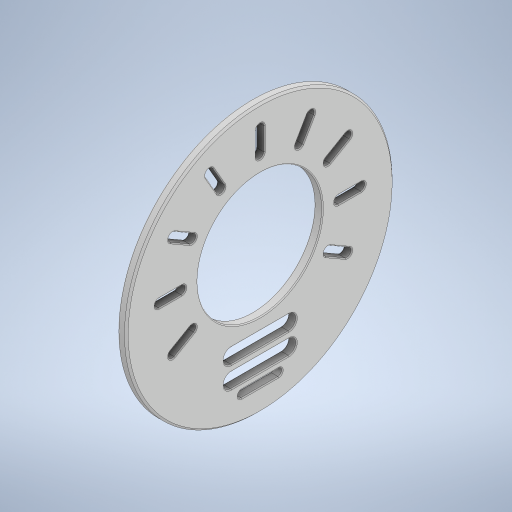
# Autodesk Inventor part: BacklightCaseFrontSymbolDisc
Saved by Autodesk Inventor 2023 (Build 270158000, 158)
## iProperties
Created: 2026-01-27
Part Number: BacklightCaseFrontSymbolDisc
Material: Generic
Document SubType Name: Modeling
Designer: DanAr
Density: 1 g/cm^3
Appearance: Default
Author: DanAr
Autodesk Inventor part; units mm, degrees
ref_plane "YZ Plane" through (0, 0, 0) normal (1, 0, 0) x (0, 1, 0)
ref_plane "XZ Plane" through (0, 0, 0) normal (0, 1, 0) x (-1, 0, 0)
ref_plane "XY Plane" through (0, 0, 0) normal (0, 0, 1) x (1, 0, 0)
sketch "Sketch1" plane through (0, 0, 0) normal (1, 0, 0) x (0, 1, 0)
  arc A0 (4.9525, -3.697) -> (-4.9525, -3.697) centre (0, 1.25) ccw
  circle A1 centre (0, 1.25) radius 6.5
  arc A2 (0.5, 12.2) -> (-0.5, 12.2) centre (0, 12.2) ccw
  arc A3 (-0.2, 9.75) -> (0.2, 9.75) centre (0, 9.75) ccw
  line L0 (0, 12.2) -> (0, 9.75) construction
  line L1 (-0.4, 12.2) -> (-0.4, 9.75)
  line L2 (0.4, 9.75) -> (0.4, 12.2)
  arc A4 (0.4, 12.2) -> (-0.4, 12.2) centre (0, 12.2) ccw
  arc A5 (-0.4, 9.75) -> (0.4, 9.75) centre (0, 9.75) ccw
  arc A6 (4.7402, -3.485) -> (-4.7403, -3.485) centre (0, 1.25) ccw
  circle A7 centre (0, 1.25) radius 10.95
  circle A8 centre (0, 1.25) radius 8.5
  circle A9 centre (0, 1.25) radius 11.35
  arc A10 (-5.3018, 10.833) -> (-5.6482, 10.633) centre (-5.475, 10.733) ccw
  arc A11 (-4.4232, 8.5112) -> (-4.0768, 8.7112) centre (-4.25, 8.6112) ccw
  line L3 (-5.475, 10.733) -> (-4.25, 8.6112) construction
  line L4 (-5.8214, 10.533) -> (-4.5964, 8.4112)
  line L5 (-3.9036, 8.8112) -> (-5.1286, 10.933)
  arc A12 (-5.1286, 10.933) -> (-5.8214, 10.533) centre (-5.475, 10.733) ccw
  arc A13 (-4.5964, 8.4112) -> (-3.9036, 8.8112) centre (-4.25, 8.6112) ccw
  arc A14 (-9.383, 6.8982) -> (-9.583, 6.5518) centre (-9.483, 6.725) ccw
  arc A15 (-7.4612, 5.3268) -> (-7.2612, 5.6732) centre (-7.3612, 5.5) ccw
  line L6 (-9.483, 6.725) -> (-7.3612, 5.5) construction
  line L7 (-9.683, 6.3786) -> (-7.5612, 5.1536)
  line L8 (-7.1612, 5.8464) -> (-9.283, 7.0714)
  arc A16 (-9.283, 7.0714) -> (-9.683, 6.3786) centre (-9.483, 6.725) ccw
  arc A17 (-7.5612, 5.1536) -> (-7.1612, 5.8464) centre (-7.3612, 5.5) ccw
  arc A18 (-10.95, 1.45) -> (-10.95, 1.05) centre (-10.95, 1.25) ccw
  arc A19 (-8.5, 1.05) -> (-8.5, 1.45) centre (-8.5, 1.25) ccw
  line L9 (-10.95, 1.25) -> (-8.5, 1.25) construction
  line L10 (-10.95, 0.85) -> (-8.5, 0.85)
  line L11 (-8.5, 1.65) -> (-10.95, 1.65)
  arc A20 (-10.95, 1.65) -> (-10.95, 0.85) centre (-10.95, 1.25) ccw
  arc A21 (-8.5, 0.85) -> (-8.5, 1.65) centre (-8.5, 1.25) ccw
  arc A22 (-7.2612, -3.1732) -> (-7.4612, -2.8268) centre (-7.3612, -3) ccw
  arc A23 (-9.583, -4.0518) -> (-9.383, -4.3982) centre (-9.483, -4.225) ccw
  line L12 (-7.3612, -3) -> (-9.483, -4.225) construction
  line L13 (-7.5612, -2.6536) -> (-9.683, -3.8786)
  line L14 (-9.283, -4.5714) -> (-7.1612, -3.3464)
  arc A24 (-7.1612, -3.3464) -> (-7.5612, -2.6536) centre (-7.3612, -3) ccw
  arc A25 (-9.683, -3.8786) -> (-9.283, -4.5714) centre (-9.483, -4.225) ccw
  arc A26 (4.0768, 8.7112) -> (4.4232, 8.5112) centre (4.25, 8.6112) ccw
  arc A27 (5.6482, 10.633) -> (5.3018, 10.833) centre (5.475, 10.733) ccw
  line L15 (4.25, 8.6112) -> (5.475, 10.733) construction
  line L16 (4.5964, 8.4112) -> (5.8214, 10.533)
  line L17 (5.1286, 10.933) -> (3.9036, 8.8112)
  arc A28 (3.9036, 8.8112) -> (4.5964, 8.4112) centre (4.25, 8.6112) ccw
  arc A29 (5.8214, 10.533) -> (5.1286, 10.933) centre (5.475, 10.733) ccw
  arc A30 (7.2612, 5.6732) -> (7.4612, 5.3268) centre (7.3612, 5.5) ccw
  arc A31 (9.583, 6.5518) -> (9.383, 6.8982) centre (9.483, 6.725) ccw
  line L18 (7.3612, 5.5) -> (9.483, 6.725) construction
  line L19 (7.5612, 5.1536) -> (9.683, 6.3786)
  line L20 (9.283, 7.0714) -> (7.1612, 5.8464)
  arc A32 (7.1612, 5.8464) -> (7.5612, 5.1536) centre (7.3612, 5.5) ccw
  arc A33 (9.683, 6.3786) -> (9.283, 7.0714) centre (9.483, 6.725) ccw
  arc A34 (8.5, 1.75) -> (8.5, 0.75) centre (8.5, 1.25) ccw
  arc A35 (10.95, 0.75) -> (10.95, 1.75) centre (10.95, 1.25) ccw
  line L21 (8.5, 1.25) -> (10.95, 1.25) construction
  line L22 (8.5, 0.85) -> (10.95, 0.85)
  line L23 (10.95, 1.65) -> (8.5, 1.65)
  arc A36 (8.5, 1.65) -> (8.5, 0.85) centre (8.5, 1.25) ccw
  arc A37 (10.95, 0.85) -> (10.95, 1.65) centre (10.95, 1.25) ccw
  arc A38 (7.4612, -2.8268) -> (7.2612, -3.1732) centre (7.3612, -3) ccw
  arc A39 (9.383, -4.3982) -> (9.583, -4.0518) centre (9.483, -4.225) ccw
  line L24 (7.3612, -3) -> (9.483, -4.225) construction
  line L25 (7.1612, -3.3464) -> (9.283, -4.5714)
  line L26 (9.683, -3.8786) -> (7.5612, -2.6536)
  arc A40 (7.5612, -2.6536) -> (7.1612, -3.3464) centre (7.3612, -3) ccw
  arc A41 (9.283, -4.5714) -> (9.683, -3.8786) centre (9.483, -4.225) ccw
  arc A42 (-3.125, -6.95) -> (-3.125, -8.25) centre (-3.125, -7.6) ccw
  arc A43 (3.125, -8.25) -> (3.125, -6.95) centre (3.125, -7.6) ccw
  line L27 (-3.125, -7.6) -> (3.125, -7.6) construction
  line L28 (-3.125, -8.25) -> (3.125, -8.25)
  line L29 (3.125, -6.95) -> (-3.125, -6.95)
  arc A44 (-3.125, -6.95) -> (-3.125, -8.25) centre (-3.125, -7.6) ccw
  arc A45 (3.125, -8.25) -> (3.125, -6.95) centre (3.125, -7.6) ccw
  arc A46 (3.125, -10.55) -> (3.125, -9.25) centre (3.125, -9.9) ccw
  arc A47 (-3.125, -9.25) -> (-3.125, -10.55) centre (-3.125, -9.9) ccw
  line L30 (3.125, -9.9) -> (-3.125, -9.9) construction
  line L31 (3.125, -9.25) -> (-3.125, -9.25)
  line L32 (-3.125, -10.55) -> (3.125, -10.55)
  arc A48 (3.125, -10.55) -> (3.125, -9.25) centre (3.125, -9.9) ccw
  arc A49 (-3.125, -9.25) -> (-3.125, -10.55) centre (-3.125, -9.9) ccw
  line L33 (2.7516, -11.25) -> (-2.7516, -11.25)
  line L34 (0, -11.25) -> (0, -12.2)
  line L35 (2.175, -12.2) -> (-2.175, -12.2)
  line L36 (2, -11.725) -> (-2, -11.725) construction
  line L37 (2, -12.025) -> (-2, -12.025)
  line L38 (-2, -11.425) -> (2, -11.425)
  arc A50 (2, -12.025) -> (2, -11.425) centre (2, -11.725) ccw
  arc A51 (-2, -11.425) -> (-2, -12.025) centre (-2, -11.725) ccw
  circle A52 centre (0, 0) radius 15
  point P0 (0, 10.975)
  point P1 (-4.8625, 9.6721)
  point P2 (-8.4221, 6.1125)
  point P3 (-9.725, 1.25)
  point P4 (-8.4221, -3.6125)
  point P5 (4.8625, 9.6721)
  point P6 (8.4221, 6.1125)
  point P7 (9.725, 1.25)
  point P8 (8.4221, -3.6125)
  point P9 (0, -7.6)
  point P10 (0, -9.9)
  point P11 (0, -11.725)
  dimension "d3" = 17
  dimension "d4" = 21.9
  dimension "d0" = 13
  dimension "d1" = 0.4
  dimension "d2" = 0.4
  dimension "d5" = 22.7
  dimension "d6" = 4
  dimension "d7" = 0.3
  dimension "d8" = 30
  constraints: 102 end point, 96 point on circle, 51 centre point, 48 tangent, 15 midpoint, 15 parallel, 4 coincident, 3 perpendicular, 2 vertical alignment, 1 collinear, 4 other
  measures "d0" diameter of A1
  measures "d1" radius of A4
  measures "d2" radius of A12
  measures "d5" diameter of A9
  measures "d6" distance of L36.start L36.end
  measures "d7" radius of A51
  measures "d8" diameter of A52
extrude "Extrusion1" add sketch "Sketch1" along normal blind 0.9 contours A9 A2 | A9 A29 L17 A7 L2 A4 | A9 A4 L1 A7 L5 A12 | A9 A33 L20 A7 L16 A29 | A12 L4 A7 L8 A16 A9 | A9 A37 L23 A7 L19 A33 | A16 L7 A7 L11 A20 A9 | A35 A9 | A7 L20 A32 A8 A28 L16 | L17 A28 A8 A5 L2 A7 | L1 A5 A8 A13 L5 A7 | A20 L10 A7 L13 A25 A9 | L4 A13 A8 A17 L8 A7 | A9 A41 L26 A7 L22 A37 | A7 L23 A36 A8 A32 L19 | A25 L14 A7 L31 A47 A9 | L7 A17 A8 A21 L11 A7 | A9 A46 L31 A7 L25 A41 | A8 A32 A34 A40 L29 A24 A21 A17 A13 A5 A28 | L10 A21 A8 A24 L13 A7 | A7 L26 A40 A8 A36 L22 | L14 A24 A8 L29 A42 L28 A43 A40 L25 A7 L31 | A36 A8 A34 | A52
sketch "Sketch2" plane through (0.9, 0, 0) normal (1, 0, 0) x (0, 0, -1)
  circle A0 centre (-1.25, 0) radius 6.5 projected
  circle A1 centre (-1.25, 0) radius 6.75
  arc A2 (-10.933, -5.1286) -> (-10.533, -5.8214) centre (-10.733, -5.475) ccw projected
  arc A3 (-8.4112, -4.5964) -> (-8.8112, -3.9036) centre (-8.6112, -4.25) ccw projected
  line L0 (-10.733, -5.475) -> (-8.6112, -4.25) construction
  line L1 (-10.508, -5.8647) -> (-8.3862, -4.6397)
  line L2 (-8.8362, -3.8603) -> (-10.958, -5.0853)
  arc A4 (-10.958, -5.0853) -> (-10.508, -5.8647) centre (-10.733, -5.475) ccw
  arc A5 (-8.3862, -4.6397) -> (-8.8362, -3.8603) centre (-8.6112, -4.25) ccw
  arc A6 (-5.1536, -7.5612) -> (-5.8464, -7.1612) centre (-5.5, -7.3612) ccw projected
  arc A7 (-7.0714, -9.283) -> (-6.3786, -9.683) centre (-6.725, -9.483) ccw projected
  line L3 (-5.5, -7.3612) -> (-6.725, -9.483) construction
  line L4 (-5.8899, -7.1361) -> (-7.1149, -9.2579)
  line L5 (-6.3351, -9.7081) -> (-5.1101, -7.5863)
  arc A8 (-5.1101, -7.5863) -> (-5.8899, -7.1361) centre (-5.5, -7.3612) ccw
  arc A9 (-7.1149, -9.2579) -> (-6.3351, -9.7081) centre (-6.725, -9.483) ccw
  arc A10 (-0.85, -8.5) -> (-1.65, -8.5) centre (-1.25, -8.5) ccw projected
  arc A11 (-1.65, -10.95) -> (-0.85, -10.95) centre (-1.25, -10.95) ccw projected
  line L6 (-1.25, -8.5) -> (-1.25, -10.95) construction
  line L7 (-1.7, -8.5) -> (-1.7, -10.95)
  line L8 (-0.8, -10.95) -> (-0.8, -8.5)
  arc A12 (-0.8, -8.5) -> (-1.7, -8.5) centre (-1.25, -8.5) ccw
  arc A13 (-1.7, -10.95) -> (-0.8, -10.95) centre (-1.25, -10.95) ccw
  arc A14 (3.3464, -7.1612) -> (2.6536, -7.5612) centre (3, -7.3612) ccw projected
  arc A15 (3.8786, -9.683) -> (4.5714, -9.283) centre (4.225, -9.483) ccw projected
  line L9 (3, -7.3612) -> (4.225, -9.483) construction
  line L10 (2.6103, -7.5862) -> (3.8353, -9.708)
  line L11 (4.6147, -9.258) -> (3.3897, -7.1362)
  arc A16 (3.3897, -7.1362) -> (2.6103, -7.5862) centre (3, -7.3612) ccw
  arc A17 (3.8353, -9.708) -> (4.6147, -9.258) centre (4.225, -9.483) ccw
  arc A18 (2.6536, 7.5612) -> (3.3464, 7.1612) centre (3, 7.3612) ccw projected
  arc A19 (4.5714, 9.283) -> (3.8786, 9.683) centre (4.225, 9.483) ccw projected
  line L12 (3, 7.3612) -> (4.225, 9.483) construction
  line L13 (3.3897, 7.1362) -> (4.6147, 9.258)
  line L14 (3.8353, 9.708) -> (2.6103, 7.5862)
  arc A20 (2.6103, 7.5862) -> (3.3897, 7.1362) centre (3, 7.3612) ccw
  arc A21 (4.6147, 9.258) -> (3.8353, 9.708) centre (4.225, 9.483) ccw
  arc A22 (-1.65, 8.5) -> (-0.85, 8.5) centre (-1.25, 8.5) ccw projected
  arc A23 (-0.85, 10.95) -> (-1.65, 10.95) centre (-1.25, 10.95) ccw projected
  line L15 (-1.25, 8.5) -> (-1.25, 10.95) construction
  line L16 (-0.8, 8.5) -> (-0.8, 10.95)
  line L17 (-1.7, 10.95) -> (-1.7, 8.5)
  arc A24 (-1.7, 8.5) -> (-0.8, 8.5) centre (-1.25, 8.5) ccw
  arc A25 (-0.8, 10.95) -> (-1.7, 10.95) centre (-1.25, 10.95) ccw
  arc A26 (-5.8464, 7.1612) -> (-5.1536, 7.5612) centre (-5.5, 7.3612) ccw projected
  arc A27 (-6.3786, 9.683) -> (-7.0714, 9.283) centre (-6.725, 9.483) ccw projected
  line L18 (-5.5, 7.3612) -> (-6.725, 9.483) construction
  line L19 (-5.1103, 7.5862) -> (-6.3353, 9.708)
  line L20 (-7.1147, 9.258) -> (-5.8897, 7.1362)
  arc A28 (-5.8897, 7.1362) -> (-5.1103, 7.5862) centre (-5.5, 7.3612) ccw
  arc A29 (-6.3353, 9.708) -> (-7.1147, 9.258) centre (-6.725, 9.483) ccw
  arc A30 (-8.8112, 3.9036) -> (-8.4112, 4.5964) centre (-8.6112, 4.25) ccw projected
  arc A31 (-10.533, 5.8214) -> (-10.933, 5.1286) centre (-10.733, 5.475) ccw projected
  line L21 (-8.6112, 4.25) -> (-10.733, 5.475) construction
  line L22 (-8.3862, 4.6397) -> (-10.508, 5.8647)
  line L23 (-10.958, 5.0853) -> (-8.8362, 3.8603)
  arc A32 (-8.8362, 3.8603) -> (-8.3862, 4.6397) centre (-8.6112, 4.25) ccw
  arc A33 (-10.508, 5.8647) -> (-10.958, 5.0853) centre (-10.733, 5.475) ccw
  arc A34 (-9.75, -0.4) -> (-9.75, 0.4) centre (-9.75, 0) ccw projected
  arc A35 (-12.2, 0.4) -> (-12.2, -0.4) centre (-12.2, 0) ccw projected
  line L24 (-9.75, 0) -> (-12.2, 0) construction
  line L25 (-9.75, 0.45) -> (-12.2, 0.45)
  line L26 (-12.2, -0.45) -> (-9.75, -0.45)
  arc A36 (-9.75, -0.45) -> (-9.75, 0.45) centre (-9.75, 0) ccw
  arc A37 (-12.2, 0.45) -> (-12.2, -0.45) centre (-12.2, 0) ccw
  arc A38 (6.95, -3.125) -> (8.25, -3.125) centre (7.6, -3.125) ccw projected
  arc A39 (8.25, 3.125) -> (6.95, 3.125) centre (7.6, 3.125) ccw projected
  line L27 (7.6, -3.125) -> (7.6, 3.125) construction
  line L28 (8.4, -3.125) -> (8.4, 3.125)
  line L29 (6.8, 3.125) -> (6.8, -3.125)
  arc A40 (6.8, -3.125) -> (8.4, -3.125) centre (7.6, -3.125) ccw
  arc A41 (8.4, 3.125) -> (6.8, 3.125) centre (7.6, 3.125) ccw
  arc A42 (9.25, -3.125) -> (10.55, -3.125) centre (9.9, -3.125) ccw projected
  arc A43 (10.55, 3.125) -> (9.25, 3.125) centre (9.9, 3.125) ccw projected
  line L30 (9.9, -3.125) -> (9.9, 3.125) construction
  line L31 (10.7, -3.125) -> (10.7, 3.125)
  line L32 (9.1, 3.125) -> (9.1, -3.125)
  arc A44 (9.1, -3.125) -> (10.7, -3.125) centre (9.9, -3.125) ccw
  arc A45 (10.7, 3.125) -> (9.1, 3.125) centre (9.9, 3.125) ccw
  arc A46 (11.425, -2) -> (12.025, -2) centre (11.725, -2) ccw projected
  arc A47 (12.025, 2) -> (11.425, 2) centre (11.725, 2) ccw projected
  line L33 (11.725, -2) -> (11.725, 2) construction
  line L34 (12.125, -2) -> (12.125, 2)
  line L35 (11.325, 2) -> (11.325, -2)
  arc A48 (11.325, -2) -> (12.125, -2) centre (11.725, -2) ccw
  arc A49 (12.125, 2) -> (11.325, 2) centre (11.725, 2) ccw
  point P0 (0, 0)
  point P1 (-9.6721, -4.8625)
  point P2 (-6.1125, -8.4221)
  point P3 (-1.25, -9.725)
  point P4 (3.6125, -8.4221)
  point P5 (3.6125, 8.4221)
  point P6 (-1.25, 9.725)
  point P7 (-6.1125, 8.4221)
  point P8 (-9.6721, 4.8625)
  point P9 (-10.975, 0)
  point P10 (7.6, 0)
  point P11 (9.9, 0)
  point P12 (11.725, 0)
  dimension "d11" = 13.5
  dimension "d12" = 0.45
  dimension "d14" = 0.8
  dimension "d15" = 1.6
  dimension "d16" = 0.4
  constraints: 96 end point, 48 point on circle, 48 tangent, 25 centre point, 15 parallel, 12 midpoint, 3 perpendicular, 1 coincident, 1 collinear
  measures "d11" diameter of A1
  measures "d12" radius of A4
  measures "d14" radius of A41
  measures "d15" distance between parallel lines of L28 L29
  measures "d16" radius of A49
extrude "Extrusion2" cut sketch "Sketch2" against normal blind 0.9 contours A0 | A1 | A4 L2 A5 L1 | A8 L5 A9 L4 | A12 L8 A13 L7 | A16 L11 A17 L10 | A20 L14 A21 L13 | A24 L17 A25 L16 | A28 L20 A29 L19 | A32 L23 A33 L22 | A36 L26 A37 L25 | A40 L29 A41 L28 | A44 L32 A45 L31 | A48 L35 A49 L34
sketch "Sketch3" plane through (0.9, 0, 0) normal (1, 0, 0) x (0, 0, -1)
  circle A0 centre (0, 0) radius 15 projected
  circle A1 centre (0, 0) radius 15
  circle A2 centre (0, 0) radius 14.5
  dimension "d19" = 29
  dimension "d20" = 30
  constraints: 2 centre point, 2 coincident
  measures "d19" diameter of A2
  measures "d20" diameter of A1
extrude "Extrusion3" cut sketch "Sketch3" against normal blind 0.9
fillet "Fillet1" radius 0.1 99 edges at (0, 0, 14.5) (0.9, 8.05, 1.25) (0.9, 9.725, 1.7) (0.9, 11.4, 1.25) (0.9, 9.725, 0.8) (0.9, 9.8727, -4.45) (0.9, 8.1971, -4.0022) (0.9, 6.9715, -2.775) (0.9, 8.6471, -3.2228) (0, 6.9715, -2.775) (0, 8.1971, -4.0022) (0, 9.8727, -4.45) (0, 8.6471, -3.2228) (0, 8.05, 1.25) (0, 9.725, 0.8) (0, 11.4, 1.25) (0, 9.725, 1.7) (0, 9.8727, 6.95) (0, 8.1971, 6.5022) (0, 6.9715, 5.275) (0, 8.6471, 5.7228) (0.9, 6.9715, 5.275) (0.9, 8.1971, 6.5022) (0.9, 9.8727, 6.95) (0.9, 8.6471, 5.7228) (0, 5.2522, 9.4471) (0, 5.7, 11.1227) (0, 4.4728, 9.8971) (0, 4.025, 8.2215) (0.9, 4.025, 8.2215) (0.9, 4.4728, 9.8971) (0.9, 5.7, 11.1227) (0.9, 5.2522, 9.4471) (0, 0, 12.65) (0, -0.45, 10.975) (0, 0, 9.3) (0, 0.45, 10.975) (0.9, 0, 9.3) (0.9, -0.45, 10.975) (0.9, 0, 12.65) (0.9, 0.45, 10.975) (0, -5.7, 11.1227) (0, -5.2522, 9.4471) (0, -4.025, 8.2215) (0, -4.4728, 9.8971) (0.9, -4.025, 8.2215) (0.9, -5.2522, 9.4471) (0.9, -5.7, 11.1227) (0.9, -4.4728, 9.8971) (0, -8.197, 6.5024) (0, -9.8728, 6.9501) (0, -8.6472, 5.7226) (0, -6.9713, 5.2749) (0.9, -8.6472, 5.7226) (0.9, -9.8728, 6.9501) (0.9, -8.197, 6.5024) (0.9, -6.9713, 5.2749) (0, -9.725, 1.7) (0, -11.4, 1.25) (0, -9.725, 0.8) (0, -8.05, 1.25) (0.9, -9.725, 0.8) (0.9, -11.4, 1.25) (0.9, -9.725, 1.7) (0.9, -8.05, 1.25) (0, -8.1971, -4.0022) (0, -6.9715, -2.775) (0, -8.6471, -3.2228) (0, -9.8727, -4.45) (0.9, -9.8727, -4.45) (0.9, -8.6471, -3.2228) (0.9, -6.9715, -2.775) (0.9, -8.1971, -4.0022) (0.9, 0, 8) (0, 0, 8) (0, 3.925, -7.6) (0, 0, -6.8) (0, -3.925, -7.6) (0, 0, -8.4) (0.9, -3.925, -7.6) (0.9, 0, -6.8) (0.9, 3.925, -7.6) (0.9, 0, -8.4) (0, -3.925, -9.9) (0, 0, -10.7) (0, 3.925, -9.9) (0, 0, -9.1) (0.9, 3.925, -9.9) (0.9, 0, -10.7) (0.9, -3.925, -9.9) (0.9, 0, -9.1) (0, -2.4, -11.725) (0, 0, -12.125) (0, 2.4, -11.725) (0, 0, -11.325) (0.9, 2.4, -11.725) (0.9, 0, -12.125) (0.9, -2.4, -11.725) (0.9, 0, -11.325)
move faces "Rotate1" rotation origin (0, 0, 0) rotation axis (1, 0, 0) rotation angle -90 translate (0, 13.925, -7.675) faces at (0.9, 7.6139, -7.7544)
move or copy body "Rotate2" bodies to move or copy 1 copy no rotation origin (0, 0, 0) rotation axis (1, 0, 0) rotation angle -90 translate (0, -1.25, 1.25)
chamfer "Chamfer1" distance 0.2 angle 45 1 edges at (0.9, 13.25, 1.25)
body "Solid1"
